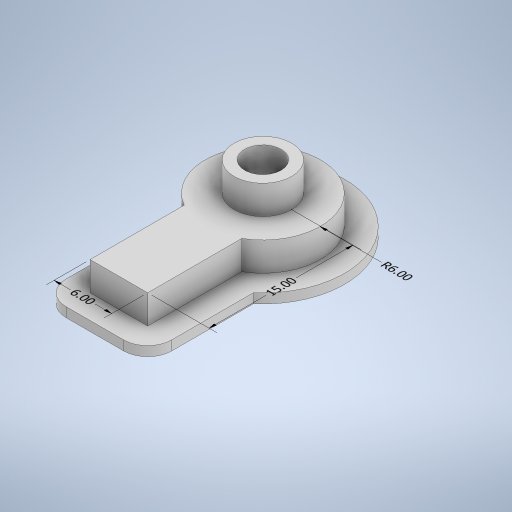
# Autodesk Inventor part: ベルト_bush_皿側
Saved by Autodesk Inventor 2024.1 (Build 281209000, 209)
## iProperties
Created: 2024-03-27
Part Number: ベルト_bush_皿側
Material: 一般
Document SubType Name: Modeling
Designer: hibik
Density: 1 g/cm^3
Appearance: 既定
Author: hibik
Autodesk Inventor part; units mm, degrees
ref_plane "YZ Plane" through (0, 0, 0) normal (1, 0, 0) x (0, 1, 0)
ref_plane "XZ Plane" through (0, 0, 0) normal (0, 1, 0) x (-1, 0, 0)
ref_plane "XY Plane" through (0, 0, 0) normal (0, 0, 1) x (1, 0, 0)
sketch "スケッチ1" plane through (0, 0, 0) normal (0, 1, 0) x (-1, 0, 0)
  circle A0 centre (0, 0) radius 6
  dimension "d0" = 12
  constraints: 1 centre point, 1 coincident
  measures "d0" diameter of A0
extrude "押し出し1" add sketch "スケッチ1" along normal blind 1
sketch "スケッチ2" plane through (0, 1, 0) normal (0, 1, 0) x (1, 0, 0)
  circle A0 centre (0, 0) radius 3
  dimension "d3" = 6
  constraints: 1 centre point, 1 coincident
  measures "d3" diameter of A0
extrude "押し出し2" add sketch "スケッチ2" along normal blind 3
sketch "スケッチ3" plane through (0, 4, 0) normal (0, 1, 0) x (1, 0, 0)
  circle A0 centre (0, 0) radius 1.9
  dimension "d6" = 3.8
  constraints: 1 centre point, 1 coincident
  measures "d6" diameter of A0
extrude "押し出し3" cut sketch "スケッチ3" against normal through all
sketch "スケッチ5" plane through (0, 1, 0) normal (0, 1, 0) x (1, 0, 0)
  circle A0 centre (0, 0) radius 3 projected
  circle A1 centre (0, 0) radius 6 projected
  line L0 (-3, 0) -> (3, 0)
  line L1 (3, 0) -> (3, -15)
  line L2 (3, -15) -> (-3, -15)
  line L3 (-3, -15) -> (-3, 0)
  circle A2 centre (0, 0) radius 3 projected
  circle A3 centre (0, 0) radius 1.9 projected
  point P0 (3, -5.1962)
  point P1 (-3, -5.1962)
  dimension "d9" = 15
  constraints: 8 end point, 2 horizontal alignment, 2 parallel, 2 vertical, 1 horizontal, 1 perpendicular, 1 other
  measures "d9" distance of L2.end L0.start
extrude "押し出し4" add sketch "スケッチ5" against normal blind 3 contours L0 A3 A0 | L1 A1 L3 A0 | A0 L0 A3 | A0 L3 A1 L1 | L1 L2 L3 A1
sketch "スケッチ6" plane through (0, -2, 0) normal (0, -1, 0) x (1, 0, 0)
  line L0 (5.5, 17.5) -> (-5.5, 17.5)
  line L1 (-5.5, 17.5) -> (-5.5, 0)
  line L2 (-5.5, 0) -> (5.5, 0)
  line L3 (5.5, 0) -> (5.5, 17.5)
  line L4 (3, 5.1962) -> (3, 15) projected
  line L5 (-3, 15) -> (-3, 5.1962) projected
  line L6 (3, 15) -> (-3, 15) projected
  arc A0 (-3, 5.1962) -> (3, 5.1962) centre (0, 0) ccw projected
  circle A1 centre (0, 0) radius 8.5
  circle A2 centre (0, 0) radius 1.9 projected
  line L7 (-6, -6.0208) -> (-6, 6.0208)
  point P0 (-5.5, 6.4807)
  point P1 (5.5, 6.4807)
  dimension "d12" = 2.5
  dimension "d13" = 2.5
  dimension "d14" = 2.5
  dimension "d15" = 2.5
  constraints: 10 end point, 2 parallel, 2 point on circle, 1 centre point, 1 coincident, 1 horizontal, 1 midpoint, 1 perpendicular, 1 tangent, 1 vertical
  measures "d12" distance between parallel lines of L3 L4
  measures "d13" distance between parallel lines of L1 L5
  measures "d14" distance between parallel lines of L6 L0
  measures "d15" radial gap between concentric circles of A1 A0
extrude "押し出し5" add sketch "スケッチ6" along normal blind 1 contours L3 A1 L4 L6 L5 L1 L0 | A1 L7 A0 L3 | L3 A0 L4 A1 | A1 L5 A0 L1 | L1 A0 L7 A1 | A0 L1 L2 A2 L3 | L3 L2 A2 L1 A0 L5 A1 L4 | A1 L5 L6 L4
fillet "フィレット1" radius 2.5 4 edges at (5.5, -2.5, 17.5) (-5.5, -2.5, 17.5) (-6, -2.5, 6.0208) (-6, -2.5, -6.0208)
